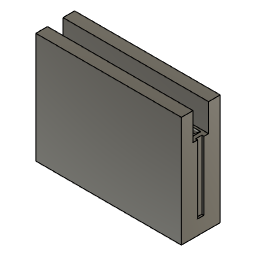
LedTaster_4TE_Stapelleistenfixierer (Autodesk Fusion 360 design; units mm, degrees)
Autodesk Fusion 360 part; units mm, degrees
sketch "Sketch1" plane through (0, 0, 0) normal (0, 0, 1) x (1, 0, 0)
  line L0 (0, 0) -> (15, 0) construction
  line L1 (15, 0) -> (15, 4)
  line L2 (15, 4) -> (0, 4)
  line L3 (0, 4) -> (0, 0) construction
  line L4 (0, 0) -> (0.65, 0) construction
  line L5 (0.65, 0) -> (0.65, 0.65)
  line L6 (0.65, 0.65) -> (0, 0.65)
  line L7 (0, 0.65) -> (0, 0) construction
  line L8 (0.65, -0.65) -> (0, -0.65)
  line L9 (0.65, 0) -> (0.65, -0.65)
  line L10 (-0.65, 0.65) -> (0, 0.65)
  line L11 (-0.65, 0) -> (-0.65, 0.65)
  line L12 (-0.65, 0) -> (-0.65, -0.65)
  line L13 (-0.65, -0.65) -> (0, -0.65)
  line L14 (1.89, 0) -> (1.89, 0.65)
  line L15 (1.89, 0.65) -> (2.54, 0.65)
  line L16 (3.19, 0) -> (3.19, 0.65)
  line L17 (3.19, 0.65) -> (2.54, 0.65)
  line L18 (3.19, 0) -> (3.19, -0.65)
  line L19 (3.19, -0.65) -> (2.54, -0.65)
  line L20 (1.89, 0) -> (1.89, -0.65)
  line L21 (1.89, -0.65) -> (2.54, -0.65)
  line L22 (2.54, 0) -> (17.54, 0) construction
  line L23 (4.43, 0) -> (4.43, 0.65)
  line L24 (4.43, 0.65) -> (5.08, 0.65)
  line L25 (5.73, 0) -> (5.73, 0.65)
  line L26 (5.73, 0.65) -> (5.08, 0.65)
  line L27 (5.73, 0) -> (5.73, -0.65)
  line L28 (5.73, -0.65) -> (5.08, -0.65)
  line L29 (4.43, 0) -> (4.43, -0.65)
  line L30 (4.43, -0.65) -> (5.08, -0.65)
  line L31 (5.08, 0) -> (20.08, 0) construction
  line L32 (6.97, 0) -> (6.97, 0.65)
  line L33 (6.97, 0.65) -> (7.62, 0.65)
  line L34 (8.27, 0) -> (8.27, 0.65)
  line L35 (8.27, 0.65) -> (7.62, 0.65)
  line L36 (8.27, 0) -> (8.27, -0.65)
  line L37 (8.27, -0.65) -> (7.62, -0.65)
  line L38 (6.97, 0) -> (6.97, -0.65)
  line L39 (6.97, -0.65) -> (7.62, -0.65)
  line L40 (7.62, 0) -> (22.62, 0) construction
  line L41 (9.51, 0) -> (9.51, 0.65)
  line L42 (9.51, 0.65) -> (10.16, 0.65)
  line L43 (10.81, 0) -> (10.81, 0.65)
  line L44 (10.81, 0.65) -> (10.16, 0.65)
  line L45 (10.81, 0) -> (10.81, -0.65)
  line L46 (10.81, -0.65) -> (10.16, -0.65)
  line L47 (9.51, 0) -> (9.51, -0.65)
  line L48 (9.51, -0.65) -> (10.16, -0.65)
  line L49 (10.16, 0) -> (25.16, 0) construction
  line L50 (12.05, 0) -> (12.05, 0.65)
  line L51 (12.05, 0.65) -> (12.7, 0.65)
  line L52 (13.35, 0) -> (13.35, 0.65)
  line L53 (13.35, 0.65) -> (12.7, 0.65)
  line L54 (13.35, 0) -> (13.35, -0.65)
  line L55 (13.35, -0.65) -> (12.7, -0.65)
  line L56 (12.05, 0) -> (12.05, -0.65)
  line L57 (12.05, -0.65) -> (12.7, -0.65)
  line L58 (12.7, 0) -> (27.7, 0) construction
  line L59 (14.59, 0) -> (14.59, 0.65)
  line L60 (14.59, 0.65) -> (15.24, 0.65)
  line L61 (15.89, 0) -> (15.89, 0.65)
  line L62 (15.89, 0.65) -> (15.24, 0.65)
  line L63 (15.89, 0) -> (15.89, -0.65)
  line L64 (15.89, -0.65) -> (15.24, -0.65)
  line L65 (14.59, 0) -> (14.59, -0.65)
  line L66 (14.59, -0.65) -> (15.24, -0.65)
  line L67 (15.24, 0) -> (30.24, 0) construction
  line L68 (-3.19, 0) -> (-3.19, 0.65)
  line L69 (-3.19, 0.65) -> (-2.54, 0.65)
  line L70 (-1.89, 0) -> (-1.89, 0.65)
  line L71 (-1.89, 0.65) -> (-2.54, 0.65)
  line L72 (-1.89, 0) -> (-1.89, -0.65)
  line L73 (-1.89, -0.65) -> (-2.54, -0.65)
  line L74 (-3.19, 0) -> (-3.19, -0.65)
  line L75 (-3.19, -0.65) -> (-2.54, -0.65)
  line L76 (-2.54, 0) -> (12.46, 0) construction
  line L77 (-5.73, 0) -> (-5.73, 0.65)
  line L78 (-5.73, 0.65) -> (-5.08, 0.65)
  line L79 (-4.43, 0) -> (-4.43, 0.65)
  line L80 (-4.43, 0.65) -> (-5.08, 0.65)
  line L81 (-4.43, 0) -> (-4.43, -0.65)
  line L82 (-4.43, -0.65) -> (-5.08, -0.65)
  line L83 (-5.73, 0) -> (-5.73, -0.65)
  line L84 (-5.73, -0.65) -> (-5.08, -0.65)
  line L85 (-5.08, 0) -> (9.92, 0) construction
  line L86 (-8.27, 0) -> (-8.27, 0.65)
  line L87 (-8.27, 0.65) -> (-7.62, 0.65)
  line L88 (-6.97, 0) -> (-6.97, 0.65)
  line L89 (-6.97, 0.65) -> (-7.62, 0.65)
  line L90 (-6.97, 0) -> (-6.97, -0.65)
  line L91 (-6.97, -0.65) -> (-7.62, -0.65)
  line L92 (-8.27, 0) -> (-8.27, -0.65)
  line L93 (-8.27, -0.65) -> (-7.62, -0.65)
  line L94 (-7.62, 0) -> (7.38, 0) construction
  line L95 (-10.81, 0) -> (-10.81, 0.65)
  line L96 (-10.81, 0.65) -> (-10.16, 0.65)
  line L97 (-9.51, 0) -> (-9.51, 0.65)
  line L98 (-9.51, 0.65) -> (-10.16, 0.65)
  line L99 (-9.51, 0) -> (-9.51, -0.65)
  line L100 (-9.51, -0.65) -> (-10.16, -0.65)
  line L101 (-10.81, 0) -> (-10.81, -0.65)
  line L102 (-10.81, -0.65) -> (-10.16, -0.65)
  line L103 (-10.16, 0) -> (4.84, 0) construction
  line L104 (-13.35, 0) -> (-13.35, 0.65)
  line L105 (-13.35, 0.65) -> (-12.7, 0.65)
  line L106 (-12.05, 0) -> (-12.05, 0.65)
  line L107 (-12.05, 0.65) -> (-12.7, 0.65)
  line L108 (-12.05, 0) -> (-12.05, -0.65)
  line L109 (-12.05, -0.65) -> (-12.7, -0.65)
  line L110 (-13.35, 0) -> (-13.35, -0.65)
  line L111 (-13.35, -0.65) -> (-12.7, -0.65)
  line L112 (-12.7, 0) -> (2.3, 0) construction
  line L113 (-15.89, 0) -> (-15.89, 0.65)
  line L114 (-15.89, 0.65) -> (-15.24, 0.65)
  line L115 (-14.59, 0) -> (-14.59, 0.65)
  line L116 (-14.59, 0.65) -> (-15.24, 0.65)
  line L117 (-14.59, 0) -> (-14.59, -0.65)
  line L118 (-14.59, -0.65) -> (-15.24, -0.65)
  line L119 (-15.89, 0) -> (-15.89, -0.65)
  line L120 (-15.89, -0.65) -> (-15.24, -0.65)
  line L121 (-15.24, 0) -> (-0.24, 0) construction
  line L122 (15, 0) -> (15, -4)
  line L123 (15, -4) -> (0, -4)
  line L124 (-15, 0) -> (-15, 4)
  line L125 (-15, 4) -> (0, 4)
  line L126 (-15, 0) -> (-15, -4)
  line L127 (-15, -4) -> (0, -4)
  dimension "d1" = 15
  dimension "d2" = 4
  dimension "d3" = 0.65
  dimension "d4" = 0.65
  dimension "d7" = 15.24
  dimension "d8" = 0
  dimension "d11" = -15.24
  dimension "d12" = 0
  constraint horizontal L0
  constraint vertical L1
  constraint horizontal L2
  constraint vertical L3
  constraint coincident L0.start L3.end
  constraint horizontal L4
  constraint vertical L5
  constraint horizontal L6
  constraint vertical L7
  constraint symmetric L5.start L4 L9.start
  constraint symmetric L5.end L4 L8.start
  constraint symmetric L6.end L4 L8.end
  constraint symmetric L4.end L7 L11.start
  constraint symmetric L5.end L7 L10.start
  constraint symmetric L6.end L7 L10.end
  constraint symmetric L7 L8.start L12.end
  constraint symmetric L7 L8.end L13.end
  constraint symmetric L7 L4.end L11.start
  constraint symmetric L0.end L22 L1.start
  constraint symmetric L1.end L22 L122.end
  constraint symmetric L2.end L22 L123.end
  constraint symmetric L0.end L3 L124.start
  constraint symmetric L1.end L3 L124.end
  constraint symmetric L2.end L3 L125.end
  constraint symmetric L3 L0.end L124.start
  constraint symmetric L3 L122.end L126.end
  constraint symmetric L3 L123.end L127.end
  measures "d1" distance of L0.start L0.end
  measures "d2" distance of L0.start L2.end
  measures "d3" distance of L0.start L4.end
  measures "d4" distance of L0.start L6.end
extrude "Extrude1" add sketch "Sketch1" along normal blind 22.8 contours L1 L2 L59 L60 L65 L66 L115 L116 L117 L118 L122 L123 L124 L125 L126 L127
sketch "Sketch2" plane through (0, 0, 22.8) normal (0, 0, 1) x (-1, 0, 0)
  line L0 (-12.05, 0.65) -> (-12.05, -0.65)
  line L1 (-12.05, -0.65) -> (-13.35, -0.65)
  line L2 (-13.35, -0.65) -> (-13.35, 0.65)
  line L3 (-13.35, 0.65) -> (-12.05, 0.65)
  line L4 (3.19, 0.65) -> (3.19, -0.65)
  line L5 (3.19, -0.65) -> (1.89, -0.65)
  line L6 (1.89, -0.65) -> (1.89, 0.65)
  line L7 (1.89, 0.65) -> (3.19, 0.65)
  line L8 (-9.51, 0.65) -> (-9.51, -0.65)
  line L9 (-9.51, -0.65) -> (-10.81, -0.65)
  line L10 (-10.81, -0.65) -> (-10.81, 0.65)
  line L11 (-10.81, 0.65) -> (-9.51, 0.65)
  line L12 (-6.97, 0.65) -> (-6.97, -0.65)
  line L13 (-6.97, -0.65) -> (-8.27, -0.65)
  line L14 (-8.27, -0.65) -> (-8.27, 0.65)
  line L15 (-8.27, 0.65) -> (-6.97, 0.65)
  line L16 (13.35, 0.65) -> (13.35, -0.65)
  line L17 (13.35, -0.65) -> (12.05, -0.65)
  line L18 (12.05, -0.65) -> (12.05, 0.65)
  line L19 (12.05, 0.65) -> (13.35, 0.65)
  line L20 (8.27, 0.65) -> (8.27, -0.65)
  line L21 (8.27, -0.65) -> (6.97, -0.65)
  line L22 (6.97, -0.65) -> (6.97, 0.65)
  line L23 (6.97, 0.65) -> (8.27, 0.65)
  line L24 (5.73, 0.65) -> (5.73, -0.65)
  line L25 (5.73, -0.65) -> (4.43, -0.65)
  line L26 (4.43, -0.65) -> (4.43, 0.65)
  line L27 (4.43, 0.65) -> (5.73, 0.65)
  line L28 (10.81, 0.65) -> (10.81, -0.65)
  line L29 (10.81, -0.65) -> (9.51, -0.65)
  line L30 (9.51, -0.65) -> (9.51, 0.65)
  line L31 (9.51, 0.65) -> (10.81, 0.65)
  line L32 (-4.43, 0.65) -> (-4.43, -0.65)
  line L33 (-4.43, -0.65) -> (-5.73, -0.65)
  line L34 (-5.73, -0.65) -> (-5.73, 0.65)
  line L35 (-5.73, 0.65) -> (-4.43, 0.65)
  line L36 (-1.89, 0.65) -> (-1.89, -0.65)
  line L37 (-1.89, -0.65) -> (-3.19, -0.65)
  line L38 (-3.19, -0.65) -> (-3.19, 0.65)
  line L39 (-3.19, 0.65) -> (-1.89, 0.65)
  line L40 (0.65, 0.65) -> (0.65, -0.65)
  line L41 (0.65, -0.65) -> (-0.65, -0.65)
  line L42 (-0.65, -0.65) -> (-0.65, 0.65)
  line L43 (-0.65, 0.65) -> (0.65, 0.65)
  line L44 (14.59, -0.65) -> (14.59, 0.65)
  line L45 (14.59, 0.65) -> (15, 0.65)
  line L46 (15, 0.65) -> (15, 4)
  line L47 (15, 4) -> (-15, 4)
  line L48 (-15, 4) -> (-15, 0.65)
  line L49 (-15, 0.65) -> (-14.59, 0.65)
  line L50 (-14.59, 0.65) -> (-14.59, -0.65)
  line L51 (-14.59, -0.65) -> (-15, -0.65)
  line L52 (-15, -0.65) -> (-15, -4)
  line L53 (-15, -4) -> (15, -4)
  line L54 (15, -4) -> (15, -0.65)
  line L55 (15, -0.65) -> (14.59, -0.65)
  line L56 (0, 0) -> (-15, 0) construction
  line L57 (-15, 0) -> (-15, -1.6)
  line L58 (-15, -1.6) -> (0, -1.6)
  line L59 (0, -1.6) -> (0, 0) construction
  line L60 (-15, 0) -> (-15, 1.6)
  line L61 (-15, 1.6) -> (0, 1.6)
  line L62 (15, 0) -> (15, -1.6)
  line L63 (15, -1.6) -> (0, -1.6)
  line L64 (15, 0) -> (15, 1.6)
  line L65 (15, 1.6) -> (0, 1.6)
  dimension "d15" = 1.6
  constraint horizontal L56
  constraint vertical L57
  constraint horizontal L58
  constraint vertical L59
  constraint coincident L56.start L59.end
  constraint symmetric L57.start L56 L60.start
  constraint symmetric L57.end L56 L60.end
  constraint symmetric L58.end L56 L61.end
  constraint symmetric L56.end L59 L62.start
  constraint symmetric L57.end L59 L62.end
  constraint symmetric L58.end L59 L63.end
  constraint symmetric L59 L56.end L62.start
  constraint symmetric L59 L60.end L64.end
  constraint symmetric L59 L61.end L65.end
  measures "d15" distance of L56.start L58.end
extrude "Extrude2" cut sketch "Sketch2" against normal blind 5.7 contours L44 L45 L46 L48 L49 L50 L51 L52 L54 L55 L57 L58 L60 L61 L62 L63 L64 L65
extrude "Extrude4" add sketch "Sketch1" along normal blind 3 contours L1 L59 L60 L65 L66 L122 | L1 L2 L59 L60 L65 L66 L115 L116 L117 L118 L122 L123 L124 L125 L126 L127 | L115 L116 L117 L118 L124 L126 | L5 L6 L8 L9 L10 L11 L12 L13 | L14 L15 L16 L17 L18 L19 L20 L21 | L23 L24 L25 L26 L27 L28 L29 L30 | L32 L33 L34 L35 L36 L37 L38 L39 | L41 L42 L43 L44 L45 L46 L47 L48 | L50 L51 L52 L53 L54 L55 L56 L57 | L68 L69 L70 L71 L72 L73 L74 L75 | L77 L78 L79 L80 L81 L82 L83 L84 | L86 L87 L88 L89 L90 L91 L92 L93 | L95 L96 L97 L98 L99 L100 L101 L102 | L104 L105 L106 L107 L108 L109 L110 L111
fillet "Fillet1" radius 0.5 44 edges at (-13.35, 0, 17.1) (-12.7, 0.65, 17.1) (-12.05, 0, 17.1) (-12.7, -0.65, 17.1) (-10.81, 0, 17.1) (-10.16, 0.65, 17.1) (-10.16, -0.65, 17.1) (-9.51, 0, 17.1) (-8.27, 0, 17.1) (-7.62, 0.65, 17.1) (-6.97, 0, 17.1) (-7.62, -0.65, 17.1) (-5.73, 0, 17.1) (-5.08, 0.65, 17.1) (-4.43, 0, 17.1) (-5.08, -0.65, 17.1) (-3.19, 0, 17.1) (-2.54, 0.65, 17.1) (-1.89, 0, 17.1) (-2.54, -0.65, 17.1) (-0.65, 0, 17.1) (0, 0.65, 17.1) (0.65, 0, 17.1) (0, -0.65, 17.1) (1.89, 0, 17.1) (2.54, 0.65, 17.1) (3.19, 0, 17.1) (2.54, -0.65, 17.1) (4.43, 0, 17.1) (5.08, 0.65, 17.1) (5.73, 0, 17.1) (5.08, -0.65, 17.1) (6.97, 0, 17.1) (7.62, 0.65, 17.1) (8.27, 0, 17.1) (7.62, -0.65, 17.1) (9.51, 0, 17.1) (10.16, 0.65, 17.1) (10.81, 0, 17.1) (10.16, -0.65, 17.1) (12.05, 0, 17.1) (12.7, 0.65, 17.1) (13.35, 0, 17.1) (12.7, -0.65, 17.1)
equation "d3 = d4"
